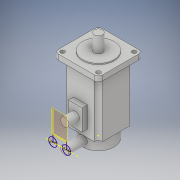
# Autodesk Inventor part: NEMA17_Stepper_CL42H60
Saved by Autodesk Inventor 2019 (Build 230136000, 136)
## iProperties
Created: 2019-08-09
Part Number: NEMA17_Stepper_CL42H60
Material: Generic
Document SubType Name: Modeling
Designer: Jorian Brusind
Density: 1 g/cm^3
Appearance: Default
Author: Jorian Brusind
Autodesk Inventor part; units mm, degrees
ref_plane "YZ Plane" through (0, 0, 0) normal (1, 0, 0) x (0, 1, 0)
ref_plane "XZ Plane" through (0, 0, 0) normal (0, 1, 0) x (-1, 0, 0)
ref_plane "XY Plane" through (0, 0, 0) normal (0, 0, 1) x (1, 0, 0)
sketch "Sketch1" plane through (0, 0, 0) normal (0, 1, 0) x (-1, 0, 0)
  line L0 (0, 0) -> (34, 0)
  line L1 (34, 0) -> (34, -34)
  line L2 (34, -34) -> (0, -34)
  line L3 (0, -34) -> (0, 0)
  dimension "d0" = 34
  dimension "d1" = 34
  constraints: 8 end point, 2 parallel, 1 horizontal, 1 perpendicular
  measures "d0" distance of L1.end L2.end
  measures "d1" distance of L0.end L1.end
extrude "Extrusion1" add sketch "Sketch1" along normal blind 54
sketch "Sketch4" plane through (0, 54, 0) normal (0, 1, 0) x (1, 0, 0)
  point P0 (0, 0)
sketch "Sketch5" plane through (0, 54, 0) normal (0, 1, 0) x (1, 0, 0)
  line L0 (-34, 34) -> (-34, 0) projected
  line L1 (0, 0) -> (-34, 0)
  line L2 (-34, 0) -> (-34, 34)
  line L3 (-34, 34) -> (0, 34)
  line L4 (0, 34) -> (0, 0)
  line L5 (4, 38) -> (-38, 38)
  line L6 (-38, 38) -> (-38, -4)
  line L7 (-38, -4) -> (4, -4)
  line L8 (4, -4) -> (4, 38)
  dimension "d15" = 4
  constraints: 16 end point, 4 parallel, 2 perpendicular, 1 horizontal, 3 other
  measures "d15" distance between parallel lines of L3 L5
extrude "Extrusion2" add sketch "Sketch5" along normal blind 5 contours L3 L4 L1 L0 | L8 L7 L6 L5
sketch "Sketch6" plane through (0, 59, 0) normal (0, 1, 0) x (1, 0, 0)
  line L0 (-34, 34) -> (-34, 0) projected
  circle A0 centre (-34, 34) radius 2
  line L1 (-38, 38) -> (-38, -4) projected
  line L2 (-38, 38) -> (-38, 34)
  line L3 (-38, 38) -> (-34, 38)
  line L4 (4, 38) -> (-38, 38) projected
  circle A1 centre (-34, 0) radius 2
  circle A2 centre (0, 34) radius 2
  circle A3 centre (0, 0) radius 2
  point P0 (0, 0)
  dimension "d18" = 4
  dimension "d21" = 34
  dimension "d24" = 34
  constraints: 4 centre point, 4 end point, 2 point on line, 1 horizontal, 1 vertical, 6 other
  measures "d18" diameter of A0
  measures "d21" distance of L0.start A1.centre
  measures "d24" distance of L0.start A2.centre
extrude "Extrusion3" cut sketch "Sketch6" against normal blind 5
sketch "Sketch8" plane through (0, 0, 0) normal (0, -1, 0) x (1, 0, 0)
  line L0 (0, -32) -> (0, -34) projected
  line L1 (0, -2) -> (0, -32) projected
  arc A0 (0, -30) -> (-4, -34) centre (0, -34) ccw
  line L2 (-32, -34) -> (-34, -34) projected
  line L3 (-34, -32) -> (-34, -2) projected
  line L4 (-34, -34) -> (-30, -34) construction
  line L5 (-34, -34) -> (-30, -34) construction
  line L6 (0, -34) -> (-4, -34)
  line L7 (-2, -34) -> (-32, -34) projected
  line L8 (0, -30) -> (0, -34)
  line L9 (-17, -34) -> (-17, -17)
  circle A1 centre (-17, -17) radius 1.5
  arc A2 (-4, 0) -> (0, -4) centre (0, 0) ccw
  line L10 (0, 0) -> (0, -4)
  line L11 (-4, 0) -> (0, 0)
  arc A3 (-34, -4) -> (-30, 0) centre (-34, 0) ccw
  line L12 (-34, 0) -> (-30, 0)
  line L13 (-34, -4) -> (-34, 0)
  arc A4 (-30, -34) -> (-34, -30) centre (-34, -34) ccw
  line L14 (-34, -34) -> (-34, -30)
  line L15 (-30, -34) -> (-34, -34)
  point P0 (0, 0)
  point P1 (0, -2)
  point P2 (-2, 0)
  point P3 (-32, 0)
  point P4 (-34, -2)
  point P5 (-34, -32)
  point P6 (-32, -34)
  dimension "d29" = 4
  dimension "d31" = 0
  dimension "d32" = 3
  dimension "d33" = 17
  dimension "d36" = 360
  constraints: 22 end point, 8 point on circle, 5 centre point, 3 collinear, 1 coincident, 1 horizontal, 1 midpoint, 1 point on line, 1 vertical, 33 other
  measures "d29" radius of A0
  measures "d31" distance between parallel lines of L4 L5
  measures "d32" diameter of A1
  measures "d33" distance from line of L7 A1.centre
extrude "Extrusion4" cut sketch "Sketch8" against normal up to surface (54 mm away) contours L0 L6 A0 L1 | L1 A2 L11 L10 | L2 L14 L3 A4 L7 | L3 L13 L12 A3
sketch "Sketch9" plane through (0, 59, 0) normal (0, 1, 0) x (1, 0, 0)
  line L0 (-38, -4) -> (4, -4) projected
  line L1 (-17, -4) -> (-17, 17)
  circle A0 centre (-17, 17) radius 15
  point P0 (0, 0)
  dimension "d40" = 21
  dimension "d41" = 30
  constraints: 2 end point, 1 centre point, 1 coincident, 1 midpoint, 1 vertical
  measures "d40" distance of L1.start L1.end
  measures "d41" diameter of A0
extrude "Extrusion5" add sketch "Sketch9" along normal blind 1
sketch "Sketch10" plane through (-17, 60, -17) normal (0, 1, 0) x (1, 0, 0)
  circle A0 centre (0, 0) radius 15 projected
  circle A1 centre (0, 0) radius 4
  line L0 (0, 0) -> (0, 3.75)
  line L1 (0, 3.75) -> (1.3919, 3.75)
  line L2 (0, 3.75) -> (-1.3919, 3.75)
  point P0 (17, -17)
  dimension "d44" = 8
  dimension "d45" = 3.75
  constraints: 6 end point, 2 point on circle, 1 centre point, 1 coincident, 1 perpendicular, 1 point on line, 1 vertical
  measures "d44" diameter of A1
  measures "d45" distance of L0.start L0.end
extrude "Extrusion6" add sketch "Sketch10" along normal blind 15 contours A1 L2 L1 picked at (-0.0068, -1.3972)
fillet "Fillet1" radius 4 4 edges at (4, 56.5, -38) (4, 56.5, 4) (-38, 56.5, -38) (-38, 56.5, 4)
sketch "Sketch11" plane through (-30, 0, 0) normal (0, 0, 1) x (1, 0, 0)
  line L0 (26, 0) -> (0, 0) projected
  line L1 (13, 0) -> (13, 17)
  line L2 (6.5, 27) -> (19.5, 27)
  line L3 (19.5, 27) -> (19.5, 7)
  line L4 (19.5, 7) -> (6.5, 7)
  line L5 (6.5, 7) -> (6.5, 27)
  line L6 (6.5, 27) -> (19.5, 7) construction
  line L7 (19.5, 27) -> (6.5, 7) construction
  point P0 (30, 0)
  dimension "d49" = 17
  dimension "d50" = 13
  dimension "d51" = 20
  constraints: 14 end point, 3 midpoint, 2 parallel, 1 horizontal, 1 perpendicular, 1 vertical
  measures "d49" distance of L1.start L1.end
  measures "d50" distance of L3.end L4.end
  measures "d51" distance of L2.end L3.end
extrude "Extrusion7" add sketch "Sketch11" along normal blind 5
ref_plane "Work Plane1" through (-30, 0, 20) normal (0, 0, 1) x (1, 0, 0)
sketch "Sketch12" plane through (-30, 0, 20) normal (0, 0, 1) x (1, 0, 0)
  line L0 (6.5, 7) -> (6.5, 27) projected
  line L1 (6.5, 7) -> (6.5, 0)
  line L2 (26, 0) -> (0, 0) projected
  circle A0 centre (6.5, 0) radius 4
  line L3 (19.5, 7) -> (6.5, 7) projected
  line L4 (19.5, 7) -> (19.5, 0)
  circle A1 centre (19.5, 0) radius 4
  point P0 (30, 0)
  dimension "d61" = 8
  dimension "d62" = 8
  constraints: 4 end point, 2 centre point, 2 coincident, 2 point on line, 2 vertical
  measures "d61" diameter of A0
  measures "d62" diameter of A1
sketch "Sketch13" plane through (0, 0, 0) normal (0, -1, 0) x (1, 0, 0)
  line L0 (0, -30) -> (0, -4) projected
  line L1 (0, -17) -> (-17, -17)
  circle A0 centre (-17, -17) radius 15
  point P0 (0, 0)
  dimension "d57" = 17
  dimension "d58" = 30
  constraints: 2 end point, 1 centre point, 1 coincident, 1 horizontal, 1 midpoint
  measures "d57" distance of L1.start L1.end
  measures "d58" diameter of A0
extrude "Extrusion8" add sketch "Sketch13" along normal blind 12
sketch "Sketch14" plane through (-23.5, 7, 0) normal (0, -1, 0) x (1, 0, 0)
  point P0 (23.5, 0)
sketch "Sketch15" plane through (-30, 0, 5) normal (0, 0, 1) x (1, 0, 0)
  line L0 (6.5, 7) -> (6.5, 27) projected
  line L1 (6.5, 17) -> (13, 17)
  circle A0 centre (13, 17) radius 4
  line L2 (13, 17) -> (13, -6)
  circle A1 centre (13, -6) radius 4
  point P0 (30, 0)
  dimension "d63" = 6.5
  dimension "d64" = 8
  dimension "d65" = 23
  dimension "d66" = 8
  constraints: 4 end point, 2 centre point, 2 coincident, 1 horizontal, 1 midpoint, 1 vertical
  measures "d63" distance of L1.start L1.end
  measures "d64" diameter of A0
  measures "d65" distance of L2.start L2.end
  measures "d66" diameter of A1
extrude "Extrusion9" add sketch "Sketch15" along normal mid plane 20
body "Solid1"
